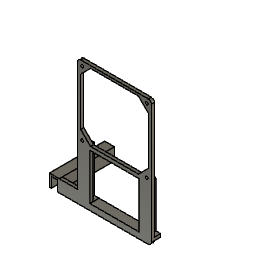
fanup v5 (Autodesk Fusion 360 design; units mm, degrees)
Autodesk Fusion 360 part; units mm, degrees
sketch "Sketch1" plane through (0, 0, 0) normal (0, 1, 0) x (1, 0, 0)
  line L0 (0, 0) -> (0, -20)
  line L1 (0, -20) -> (16, -20)
  line L2 (16, -20) -> (16, 0)
  line L3 (16, 0) -> (13, 0)
  line L4 (13, 0) -> (13, -17)
  line L5 (13, -17) -> (3, -17)
  line L6 (3, -17) -> (3, 0)
  line L7 (3, 0) -> (0, 0)
  constraint coincident L0.start L7.end
  constraint vertical L0
  constraint perpendicular L0 L1
  constraint perpendicular L1 L2
  constraint perpendicular L0 L3
  constraint perpendicular L3 L4
  constraint perpendicular L4 L5
  constraint perpendicular L5 L6
  constraint perpendicular L0 L7
extrude "Extrude1" add sketch "Sketch1" along normal blind 60
sketch "Sketch2" plane through (0, 0, 0) normal (0, -1, 0) x (1, 0, 0)
  line L0 (0, 0) -> (3, 0)
  line L1 (3, 0) -> (3, 17)
  line L2 (3, 17) -> (13, 17)
  line L3 (13, 17) -> (13, 0)
  line L4 (13, 0) -> (16, 0)
  line L5 (16, 0) -> (16, 20)
  line L6 (16, 20) -> (0, 20)
  line L7 (0, 20) -> (0, 0)
  line L8 (16, 0) -> (66, 0)
  line L9 (66, 0) -> (66, 85)
  line L10 (66, 85) -> (146, 85)
  line L11 (146, 85) -> (146, 0)
  line L12 (146, 0) -> (166, 0)
  line L13 (166, 0) -> (166, 205)
  line L14 (166, 205) -> (46, 205)
  line L15 (46, 205) -> (46, 20)
  line L16 (46, 20) -> (16, 20)
  dimension "d3" = 50
  dimension "d4" = 85
  dimension "d5" = 80
  dimension "d6" = 20
  dimension "d7" = 205
  dimension "d8" = 120
  dimension "d9" = 185
  constraint coincident L4.end L5.start
  constraint perpendicular L5 L8
  constraint perpendicular L8 L9
  constraint perpendicular L9 L10
  constraint perpendicular L8 L11
  constraint perpendicular L11 L12
  constraint perpendicular L12 L13
  constraint perpendicular L13 L14
  constraint perpendicular L14 L15
  constraint coincident L5.end L6.start
  measures "d3" distance of L4.end L8.end
  measures "d4" distance of L8.end L9.end
  measures "d5" distance of L9.end L10.end
  measures "d6" distance of L11.end L12.end
  measures "d7" distance of L12.end L13.end
  measures "d8" distance of L13.end L14.end
  measures "d9" distance of L14.end L15.end
extrude "Extrude2" add sketch "Sketch2" against normal blind 3 contours L5 L8 L9 L10 L11 L12 L13 L14 L15 L16
sketch "Sketch3" plane through (0, 0, 0) normal (0, 1, 0) x (1, 0, 0)
  line L0 (65, 0) -> (150, 0)
  line L1 (150, 0) -> (150, -10)
  line L2 (150, -10) -> (65, -10)
  line L3 (65, -10) -> (65, 0)
  constraint horizontal L0
  constraint vertical L1
  constraint horizontal L2
  constraint vertical L3
extrude "Extrude3" add sketch "Sketch3" along normal blind 3
sketch "Sketch4" plane through (0, 0, 0) normal (0, 1, 0) x (1, 0, 0)
sketch "Sketch5" plane through (0, 0, 0) normal (0, 0, 1) x (1, 0, 0)
  line L0 (16, 3) -> (16, 30)
  line L1 (16, 30) -> (43, 3)
  line L2 (43, 3) -> (16, 3)
  constraint vertical L0
  constraint perpendicular L0 L2
extrude "Extrude4" add sketch "Sketch5" along normal blind 3
sketch "Sketch6" plane through (0, 0, 0) normal (0, -1, 0) x (1, 0, 0)
  line L0 (66, 10) -> (66, 85)
  line L1 (66, 85) -> (146, 85)
  line L2 (146, 85) -> (146, 10)
  line L3 (146, 10) -> (66, 10)
  line L4 (13, 0) -> (166, 0)
  line L5 (166, 0) -> (166, 205)
  line L6 (166, 205) -> (46, 205)
  line L7 (46, 205) -> (46, 20)
  line L8 (46, 20) -> (16, 20)
  line L9 (16, 20) -> (0, 20)
  line L10 (0, 20) -> (0, 0)
  line L11 (0, 0) -> (3, 0)
  line L12 (3, 0) -> (3, 17)
  line L13 (3, 17) -> (13, 17)
  line L14 (13, 17) -> (13, 0)
  circle A0 centre (51.25, 199.75) radius 2.25
  circle A1 centre (160.75, 199.75) radius 2.25
  circle A2 centre (51.25, 90.25) radius 2.25
  circle A3 centre (160.75, 90.25) radius 2.25
  dimension "d16" = 4.5
  dimension "d17" = 5.25
  dimension "d18" = 5.25
  dimension "d19" = 4.5
  dimension "d20" = 5.25
  dimension "d21" = 5.25
  dimension "d22" = 4.5
  dimension "d23" = 5.25
  dimension "d24" = 114.75
  dimension "d25" = 4.5
  dimension "d26" = 5.25
  dimension "d27" = 114.75
  measures "d16" diameter of A0
  measures "d17" distance of L7 A0.centre
  measures "d18" distance of L6 A0.centre
  measures "d19" diameter of A1
  measures "d20" distance of L5 A1.centre
  measures "d21" distance of L6 A1.centre
  measures "d22" diameter of A2
  measures "d23" distance of L7 A2.centre
  measures "d24" distance of L6 A2.centre
  measures "d25" diameter of A3
  measures "d26" distance of L5 A3.centre
  measures "d27" distance of L6 A3.centre
extrude "Extrude5" cut sketch "Sketch6" against normal blind 5 contours A0 | A1 | A2 | A3
sketch "Sketch7" plane through (0, 0, 0) normal (0, -1, 0) x (1, 0, 0)
  circle A0 centre (160.75, 90.25) radius 2.25
  circle A1 centre (160.75, 199.75) radius 2.25
  circle A2 centre (51.25, 90.25) radius 2.25
  circle A3 centre (51.25, 199.75) radius 2.25
  line L0 (66, 10) -> (66, 85)
  line L1 (66, 85) -> (146, 85)
  line L2 (146, 85) -> (146, 10)
  line L3 (146, 10) -> (66, 10)
  line L4 (13, 0) -> (166, 0)
  line L5 (166, 0) -> (166, 205)
  line L6 (166, 205) -> (46, 205)
  line L7 (46, 205) -> (46, 20)
  line L8 (46, 20) -> (16, 20)
  line L9 (16, 20) -> (0, 20)
  line L10 (0, 20) -> (0, 0)
  line L11 (0, 0) -> (3, 0)
  line L12 (3, 0) -> (3, 17)
  line L13 (3, 17) -> (13, 17)
  line L14 (13, 17) -> (13, 0)
  line L15 (51, 185) -> (67, 201)
  line L16 (67, 201) -> (145, 201)
  line L17 (145, 201) -> (160.9711, 185.0289)
  line L18 (160.9711, 185.0289) -> (160.9711, 107.0289)
  line L19 (51, 185) -> (51, 107)
  line L20 (51, 107) -> (66.9997, 91.0003)
  line L21 (66.9997, 91.0003) -> (144.9997, 91.0003)
  line L22 (144.9997, 91.0003) -> (160.9711, 107.0289)
  dimension "d30" = 78
  dimension "d31" = 22.627
  dimension "d32" = 78
  dimension "d33" = 78
  constraint parallel L6 L16
  constraint perpendicular L15 L17
  constraint perpendicular L16 L18
  constraint parallel L7 L19
  constraint perpendicular L15 L20
  constraint horizontal L21
  measures "d30" distance of L15.start L19.end
  measures "d31" distance of L19.end L20.end
  measures "d32" distance of L17.end L18.end
  measures "d33" distance of L20.end L21.end
extrude "Extrude6" cut sketch "Sketch7" against normal blind 10 contours L15 L16 L17 L18 L19 L20 L21 L22
sketch "Sketch8" plane through (0, 0, 0) normal (0, -1, 0) x (1, 0, 0)
  line L0 (66.9997, 91.0003) -> (51, 107)
  line L1 (51, 107) -> (51, 185)
  line L2 (51, 185) -> (67, 201)
  line L3 (67, 201) -> (145, 201)
  line L4 (145, 201) -> (160.9711, 185.0289)
  line L5 (160.9711, 185.0289) -> (160.9711, 107.0289)
  line L6 (160.9711, 107.0289) -> (144.9997, 91.0003)
  line L7 (144.9997, 91.0003) -> (66.9997, 91.0003)
  circle A0 centre (160.75, 90.25) radius 2.25
  circle A1 centre (160.75, 199.75) radius 2.25
  circle A2 centre (51.25, 90.25) radius 2.25
  line L8 (66, 10) -> (66, 85)
  line L9 (66, 85) -> (146, 85)
  line L10 (146, 85) -> (146, 10)
  line L11 (146, 10) -> (66, 10)
  line L12 (13, 0) -> (166, 0)
  line L13 (166, 0) -> (166, 205)
  line L14 (166, 205) -> (46, 205)
  line L15 (46, 205) -> (46, 20)
  line L16 (46, 20) -> (16, 20)
  line L17 (16, 20) -> (0, 20)
  line L18 (0, 20) -> (0, 0)
  line L19 (0, 0) -> (3, 0)
  line L20 (3, 0) -> (3, 17)
  line L21 (3, 17) -> (13, 17)
  line L22 (13, 17) -> (13, 0)
sketch "Sketch9" plane through (0, 0, 0) normal (0, -1, 0) x (1, 0, 0)
  circle A0 centre (51, 200) radius 3.6056
extrude "Extrude7" add sketch "Sketch9" against normal blind 3
sketch "Sketch10" plane through (0, 0, 0) normal (0, -1, 0) x (1, 0, 0)
  circle A0 centre (53.5, 197.5) radius 2.25
  line L0 (46, 205) -> (46, 20)
  line L1 (166, 205) -> (46, 205)
  dimension "d38" = 4.5
  dimension "d39" = 7.5
  dimension "d40" = 7.5
  measures "d38" diameter of A0
  measures "d39" distance of A0.centre L0
  measures "d40" distance of A0.centre L1
sketch "Sketch11" plane through (0, 0, 0) normal (0, -1, 0) x (1, 0, 0)
  circle A0 centre (160, 200) radius 4.464
extrude "Extrude8" add sketch "Sketch11" against normal blind 3
sketch "Sketch12" plane through (0, 0, 0) normal (0, -1, 0) x (1, 0, 0)
  circle A0 centre (158.5, 197.5) radius 2.25
  line L0 (166, 0) -> (166, 205)
  line L1 (166, 205) -> (46, 205)
  dimension "d43" = 4.5
  dimension "d44" = 7.5
  dimension "d45" = 7.5
  measures "d43" diameter of A0
  measures "d44" distance of A0.centre L0
  measures "d45" distance of A0.centre L1
extrude "Extrude9" cut sketch "Sketch10" against normal blind 3
extrude "Extrude10" cut sketch "Sketch12" against normal blind 3
sketch "Sketch13" plane through (0, 0, 0) normal (0, -1, 0) x (1, 0, 0)
  circle A0 centre (50, 90) radius 3.5652
  circle A1 centre (160, 90) radius 4.4009
extrude "Extrude11" add sketch "Sketch13" against normal blind 3 contours A0
extrude "Extrude12" add sketch "Sketch8" against normal blind 3 contours A0
sketch "Sketch14" plane through (0, 0, 0) normal (0, -1, 0) x (1, 0, 0)
  circle A0 centre (158.5, 197.5) radius 2.25
  circle A1 centre (53.5, 197.5) radius 2.25
  line L0 (66.9997, 91.0003) -> (51, 107)
  line L1 (51, 107) -> (51, 185)
  line L2 (51, 185) -> (67, 201)
  line L3 (67, 201) -> (145, 201)
  line L4 (145, 201) -> (160.9711, 185.0289)
  line L5 (160.9711, 185.0289) -> (160.9711, 107.0289)
  line L6 (160.9711, 107.0289) -> (144.9997, 91.0003)
  line L7 (144.9997, 91.0003) -> (66.9997, 91.0003)
  line L8 (66, 10) -> (66, 85)
  line L9 (66, 85) -> (146, 85)
  line L10 (146, 85) -> (146, 10)
  line L11 (146, 10) -> (66, 10)
  line L12 (13, 0) -> (166, 0)
  line L13 (166, 0) -> (166, 205)
  line L14 (166, 205) -> (46, 205)
  line L15 (46, 205) -> (46, 20)
  line L16 (46, 20) -> (16, 20)
  line L17 (16, 20) -> (0, 20)
  line L18 (0, 20) -> (0, 0)
  line L19 (0, 0) -> (3, 0)
  line L20 (3, 0) -> (3, 17)
  line L21 (3, 17) -> (13, 17)
  line L22 (13, 17) -> (13, 0)
  circle A2 centre (53.5, 92.5) radius 2.25
  circle A3 centre (158.5, 92.5) radius 2.25
  dimension "d54" = 4.5
  dimension "d55" = 7.5
  dimension "d57" = 7.5
  dimension "d58" = 4.5
  dimension "d59" = 7.5
  dimension "d60" = 7.5
  measures "d54" diameter of A2
  measures "d55" distance of L15 A2.centre
  measures "d57" distance of L9 A2.centre
  measures "d58" diameter of A3
  measures "d59" distance of L13 A3.centre
  measures "d60" distance of L9 A3.centre
extrude "Extrude13" cut sketch "Sketch14" against normal blind 3 contours A2 | A3
fillet "Fillet1" radius 5 1 edges at (46, 1.5, 205)
fillet "Fillet2" radius 5 1 edges at (166, 1.5, 205)
fillet "Fillet3" radius 5 1 edges at (166, 1.5, 0)
extrude "Extrude14" add 1 faces at (59.3333, 3, 38.3333) along direction (0, 1, 0) blind 2
sketch "Sketch15" plane through (0, 5, 0) normal (0, 1, 0) x (-1, 0, 0)
  arc A0 (-166, 5) -> (-161, 0) centre (-161, 5) ccw
  line L0 (-161, 0) -> (-43, 0)
  line L1 (-43, 0) -> (-43, 3)
  line L2 (-43, 3) -> (-41, 3)
  line L3 (-41, 3) -> (-16, 3)
  line L4 (-16, 3) -> (-16, 20)
  line L5 (-16, 20) -> (-46, 20)
  line L6 (-46, 20) -> (-46, 200)
  arc A1 (-46, 200) -> (-51, 205) centre (-51, 200) ccw
  line L7 (-51, 205) -> (-161, 205)
  arc A2 (-161, 205) -> (-166, 200) centre (-161, 200) ccw
  line L8 (-166, 200) -> (-166, 5)
  circle A3 centre (-53.5, 92.5) radius 2.25
  circle A4 centre (-158.5, 92.5) radius 2.25
  circle A5 centre (-158.5, 197.5) radius 2.25
  circle A6 centre (-53.5, 197.5) radius 2.25
  line L9 (-51, 107) -> (-66.9997, 91.0003)
  line L10 (-66.9997, 91.0003) -> (-144.9997, 91.0003)
  line L11 (-144.9997, 91.0003) -> (-160.9711, 107.0289)
  line L12 (-160.9711, 107.0289) -> (-160.9711, 185.0289)
  line L13 (-160.9711, 185.0289) -> (-145, 201)
  line L14 (-145, 201) -> (-67, 201)
  line L15 (-67, 201) -> (-51, 185)
  line L16 (-51, 185) -> (-51, 107)
  line L17 (-66, 10) -> (-146, 10)
  line L18 (-146, 10) -> (-146, 85)
  line L19 (-146, 85) -> (-66, 85)
  line L20 (-66, 85) -> (-66, 10)
  line L21 (-166, 10.0934) -> (-16, 10.0934)
  line L22 (-16, 10.0934) -> (-16, 5.0934)
  line L23 (-16, 5.0934) -> (-166, 5.0934)
  line L24 (-166, 5.0934) -> (-166, 10.0934)
  dimension "d71" = 5
  constraint horizontal L21
  constraint vertical L22
  constraint horizontal L23
  constraint vertical L24
  constraint coincident L4 L22.end
  constraint coincident L8 L21.start
  measures "d71" distance of L21.start L23.end
extrude "Extrude15" add sketch "Sketch15" along normal blind 10 contours L4 L8 L17 L18 L20 L21 L22 L23 L24
sketch "Sketch16" plane through (0, 5, 0) normal (0, 1, 0) x (-1, 0, 0)
  line L0 (-166, 10.0934) -> (-146, 10.0934)
  line L1 (-146, 10.0934) -> (-146, 85)
  line L2 (-146, 85) -> (-66, 85)
  line L3 (-66, 85) -> (-66, 10.0934)
  line L4 (-66, 10.0934) -> (-16, 10.0934)
  line L5 (-16, 10.0934) -> (-16, 20)
  line L6 (-16, 20) -> (-46, 20)
  line L7 (-46, 20) -> (-46, 200)
  arc A0 (-46, 200) -> (-51, 205) centre (-51, 200) ccw
  line L8 (-51, 205) -> (-161, 205)
  arc A1 (-161, 205) -> (-166, 200) centre (-161, 200) ccw
  line L9 (-166, 200) -> (-166, 10.0934)
  line L10 (-51, 107) -> (-66.9997, 91.0003)
  line L11 (-66.9997, 91.0003) -> (-144.9997, 91.0003)
  line L12 (-144.9997, 91.0003) -> (-160.9711, 107.0289)
  line L13 (-160.9711, 107.0289) -> (-160.9711, 185.0289)
  line L14 (-160.9711, 185.0289) -> (-145, 201)
  line L15 (-145, 201) -> (-67, 201)
  line L16 (-67, 201) -> (-51, 185)
  line L17 (-51, 185) -> (-51, 107)
  circle A2 centre (-53.5, 197.5) radius 2.25
  circle A3 centre (-158.5, 197.5) radius 2.25
  circle A4 centre (-158.5, 92.5) radius 2.25
  circle A5 centre (-53.5, 92.5) radius 2.25
  line L18 (-158.5, 10.0934) -> (-153.5, 10.0934)
  line L19 (-153.5, 10.0934) -> (-153.5, 85.0934)
  line L20 (-153.5, 85.0934) -> (-158.5, 85.0934)
  line L21 (-158.5, 85.0934) -> (-158.5, 10.0934)
  dimension "d74" = 75
  dimension "d75" = 7.5
  dimension "d76" = 5
  constraint horizontal L18
  constraint vertical L19
  constraint horizontal L20
  constraint vertical L21
  constraint coincident L0 L18.start
  measures "d74" distance of L18.start L20.end
  measures "d75" distance of L1 L19
  measures "d76" distance of L18.start L18.end
extrude "Extrude16" add sketch "Sketch16" along normal blind 10 contours L0 L18 L19 L20 L21
sketch "Sketch17" plane through (0, 5, 0) normal (0, 1, 0) x (-1, 0, 0)
  circle A0 centre (-53.5, 92.5) radius 2.25
  circle A1 centre (-158.5, 92.5) radius 2.25
  circle A2 centre (-158.5, 197.5) radius 2.25
  circle A3 centre (-53.5, 197.5) radius 2.25
  line L0 (-51, 107) -> (-66.9997, 91.0003)
  line L1 (-66.9997, 91.0003) -> (-144.9997, 91.0003)
  line L2 (-144.9997, 91.0003) -> (-160.9711, 107.0289)
  line L3 (-160.9711, 107.0289) -> (-160.9711, 185.0289)
  line L4 (-160.9711, 185.0289) -> (-145, 201)
  line L5 (-145, 201) -> (-67, 201)
  line L6 (-67, 201) -> (-51, 185)
  line L7 (-51, 185) -> (-51, 107)
  line L8 (-158.5, 10.0934) -> (-158.5, 85.0934)
  line L9 (-158.5, 85.0934) -> (-153.5, 85.0934)
  line L10 (-153.5, 85.0934) -> (-153.5, 10.0934)
  line L11 (-153.5, 10.0934) -> (-146, 10.0934)
  line L12 (-146, 10.0934) -> (-146, 85)
  line L13 (-146, 85) -> (-66, 85)
  line L14 (-66, 85) -> (-66, 10.0934)
  line L15 (-66, 10.0934) -> (-16, 10.0934)
  line L16 (-16, 10.0934) -> (-16, 20)
  line L17 (-16, 20) -> (-46, 20)
  line L18 (-46, 20) -> (-46, 200)
  arc A4 (-46, 200) -> (-51, 205) centre (-51, 200) ccw
  line L19 (-51, 205) -> (-161, 205)
  arc A5 (-161, 205) -> (-166, 200) centre (-161, 200) ccw
  line L20 (-166, 200) -> (-166, 10.0934)
  line L21 (-166, 10.0934) -> (-158.5, 10.0934)
  line L22 (-58.5, 10.0934) -> (-53.5, 10.0934)
  line L23 (-53.5, 10.0934) -> (-53.5, 85.0934)
  line L24 (-53.5, 85.0934) -> (-58.5, 85.0934)
  line L25 (-58.5, 85.0934) -> (-58.5, 10.0934)
  dimension "d79" = 5
  dimension "d80" = 75
  dimension "d81" = 7.5
  constraint horizontal L22
  constraint vertical L23
  constraint horizontal L24
  constraint vertical L25
  constraint coincident L15 L22.start
  measures "d79" distance of L22.start L22.end
  measures "d80" distance of L22.start L24.end
  measures "d81" distance of L14 L25
extrude "Extrude17" add sketch "Sketch17" along normal blind 10 contours L15 L22 L23 L24 L25
extrude "Extrude18" add 1 faces at (1, 60, 12.3333) along direction (0, 1, 0) blind 30
